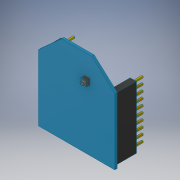
# Autodesk Inventor part: Xbee
Saved by Autodesk Inventor 2019 (Build 230136000, 136)
## iProperties
Created: 2019-08-29
Part Number: Xbee
Material: Générique
Document SubType Name: Modeling
Designer: Sébastien DI MERCURIO
Density: 1 g/cm^3
Appearance: Bleu ciel foncé
Author: Sébastien DI MERCURIO
Autodesk Inventor part; units mm, degrees
ref_plane "YZ Plane" through (0, 0, 0) normal (1, 0, 0) x (0, 1, 0)
ref_plane "XZ Plane" through (0, 0, 0) normal (0, 1, 0) x (-1, 0, 0)
ref_plane "XY Plane" through (0, 0, 0) normal (0, 0, 1) x (1, 0, 0)
sketch "Esquisse1" plane through (0, 0, 0) normal (0, 0, 1) x (1, 0, 0)
  line L0 (-12.25, -10.6) -> (12.25, -10.6)
  line L1 (12.25, -10.6) -> (12.25, 10.6)
  line L2 (12.25, 10.6) -> (4.85, 17.3)
  line L3 (4.85, 17.3) -> (-4.85, 17.3)
  line L4 (-4.85, 17.3) -> (-12.25, 10.6)
  line L5 (-12.25, 10.6) -> (-12.25, -10.6)
  point P0 (0, 0)
  dimension "d0" = 24.5
  dimension "d1" = 27.9
  dimension "d2" = 21.2
  dimension "d3" = 12.25
  dimension "d4" = 10.6
  dimension "d6" = 9.7
  constraints: 12 end point, 2 equal length, 2 parallel, 1 horizontal, 1 perpendicular
  measures "d0" distance of L0.start L0.end
  measures "d1" distance between parallel lines of L3 L0
  measures "d2" distance of L0.end L1.end
  measures "d3" horizontal distance of point (0, 0) L0.start
  measures "d4" vertical distance of L0.start point (0, 0)
  measures "d6" distance of L2.end L3.end
extrude "Extrusion1" add sketch "Esquisse1" along normal blind 0.8
sketch "Esquisse2" plane through (0, 0, 0) normal (0, 0, -1) x (-1, 0, 0)
  line L0 (12.1, 10.4) -> (10.1, 10.4)
  line L1 (10.1, 10.4) -> (10.1, -9.6)
  line L2 (10.1, -9.6) -> (12.1, -9.6)
  line L3 (12.1, -9.6) -> (12.1, 10.4)
  line L4 (-10.1, 10.4) -> (-12.1, 10.4)
  line L5 (-12.1, 10.4) -> (-12.1, -9.6)
  line L6 (-12.1, -9.6) -> (-10.1, -9.6)
  line L7 (-10.1, -9.6) -> (-10.1, 10.4)
  line L8 (12.25, -10.6) -> (-12.25, -10.6) projected
  line L9 (-12.25, -10.6) -> (-12.25, 10.6) projected
  point P0 (0, 0)
  dimension "d9" = 2
  dimension "d10" = 20.2
  dimension "d11" = 20
  dimension "d12" = 1
  dimension "d13" = 24.2
  dimension "d14" = 0.15
  dimension "d15" = 24.5
  constraints: 16 end point, 4 parallel, 2 equal length, 2 horizontal, 2 perpendicular, 1 collinear
  measures "d9" distance of L1.end L2.end
  measures "d10" distance between parallel lines of L7 L1
  measures "d11" distance of L4.end L5.end
  measures "d12" distance between parallel lines of L8 L2
  measures "d13" distance between parallel lines of L5 L3
  measures "d14" distance from line of L9 L5.end
  measures "d15" distance of L8.start L8.end
extrude "Extrusion2" add sketch "Esquisse2" along normal blind 6.3
sketch "Esquisse3" plane through (0, 0, -6.3) normal (0, 0, -1) x (-1, 0, 0)
  line L0 (11.2482, 9.9) -> (10.7482, 9.9)
  line L1 (10.7482, 9.9) -> (10.7482, 9.4)
  line L2 (10.7482, 9.4) -> (11.2482, 9.4)
  line L3 (11.2482, 9.4) -> (11.2482, 9.9)
  line L4 (-10.7482, 9.9) -> (-11.2482, 9.9)
  line L5 (-11.2482, 9.9) -> (-11.2482, 9.4)
  line L6 (-11.2482, 9.4) -> (-10.7482, 9.4)
  line L7 (-10.7482, 9.4) -> (-10.7482, 9.9)
  line L8 (10.1, 10.4) -> (10.1, -9.6) projected
  line L9 (12.1, -9.6) -> (12.1, 10.4) projected
  line L10 (-12.25, -10.6) -> (-12.25, 10.6) projected
  line L11 (12.25, 10.6) -> (12.25, -10.6) projected
  line L12 (12.1, 10.4) -> (10.1, 10.4) projected
  point P0 (0, 0)
  dimension "d18" = 2
  dimension "d19" = 21.4964
  dimension "d20" = 0.5
  dimension "d21" = 24.5
  dimension "d22" = 1.5018
  dimension "d23" = 0.5
  constraints: 16 end point, 4 parallel, 2 equal length, 2 horizontal, 2 perpendicular, 2 point on line
  measures "d18" distance between parallel lines of L8 L9
  measures "d19" distance between parallel lines of L7 L1
  measures "d20" distance of L2.end L0.start
  measures "d21" distance between parallel lines of L10 L11
  measures "d22" distance between parallel lines of L11 L1
  measures "d23" distance between parallel lines of L12 L0
extrude "Extrusion3" add sketch "Esquisse3" along normal blind 3.2
chamfer "Chanfrein1" distance 0.15 angle 45 4 edges at (-10.7482, 9.65, -9.5) (-10.9982, 9.9, -9.5) (-11.2482, 9.65, -9.5) (-10.9982, 9.4, -9.5)
chamfer "Chanfrein2" distance 0.15 angle 45 4 edges at (10.9982, 9.9, -9.5) (10.9982, 9.4, -9.5) (11.2482, 9.65, -9.5) (10.7482, 9.65, -9.5)
pattern_linear "Réseau rectangulaire1" count 10 spacing 2 along (0, -1, 0) of "Extrusion3", "Chanfrein1", "Chanfrein2"
sketch "Esquisse4" plane through (0, 0, 0.8) normal (0, 0, 1) x (1, 0, 0)
  line L0 (2.55, 9) -> (4.25, 9)
  line L1 (4.25, 9) -> (4.25, 10.8)
  line L2 (4.25, 10.8) -> (2.55, 10.8)
  line L3 (2.55, 10.8) -> (2.55, 9)
  line L4 (4.85, 17.3) -> (-4.85, 17.3) projected
  line L5 (12.25, -10.6) -> (12.25, 10.6) projected
  point P0 (0, 0)
  dimension "d35" = 1.8
  dimension "d36" = 1.7
  dimension "d37" = 6.5
  dimension "d38" = 8
  constraints: 8 end point, 2 parallel, 1 horizontal, 1 perpendicular
  measures "d35" distance of L2.end L0.start
  measures "d36" distance of L1.end L2.end
  measures "d37" distance between parallel lines of L4 L2
  measures "d38" distance between parallel lines of L5 L1
extrude "Extrusion4" add sketch "Esquisse4" along normal blind 1.2
sketch "Esquisse5" plane through (0, 0, 2) normal (0, 0, 1) x (1, 0, 0)
  circle A0 centre (3.4, 9.9) radius 0.65
  circle A1 centre (3.4, 9.9) radius 0.4
  line L0 (2.55, 10.8) -> (2.55, 9) projected
  line L1 (2.55, 9) -> (4.25, 9) projected
  point P0 (0, 0)
  dimension "d41" = 1.3
  dimension "d42" = 0.8
  dimension "d43" = 0.85
  dimension "d44" = 0.9
  constraints: 2 centre point, 1 coincident
  measures "d41" diameter of A0
  measures "d42" diameter of A1
  measures "d43" distance from line of L0 A0.centre
  measures "d44" distance from line of L1 A0.centre
extrude "Extrusion5" add sketch "Esquisse5" along normal blind 0.5
equation "\"d3\" = 0.5 * d0"
equation "\"d4\" = 0.5 * d2"
equation "\"d14\" = -0.5 * d13 + 0.5 * d15"
equation "\"d22\" = -0.5 * d19 + 0.5 * d21"
